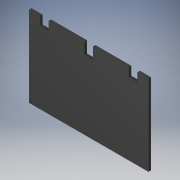
# Autodesk Inventor part: BA12
Saved by Autodesk Inventor 2017 (Build 210142000, 142)
## iProperties
Created: 2018-10-18
Part Number: BA12
Material: ABS Plastic
Document SubType Name: Modeling
Designer: Dell
Density: 1.06 g/cm^3
Appearance: Smooth - Black
Author: Dell
Autodesk Inventor part; units mm, degrees
ref_plane "YZ Plane" through (0, 0, 0) normal (1, 0, 0) x (0, 1, 0)
ref_plane "XZ Plane" through (0, 0, 0) normal (0, 1, 0) x (-1, 0, 0)
ref_plane "XY Plane" through (0, 0, 0) normal (0, 0, 1) x (1, 0, 0)
sketch "Sketch1" plane through (0, 0, 0) normal (0, 0, 1) x (1, 0, 0)
  line L0 (0, 0) -> (262.89, 0)
  line L1 (262.89, 0) -> (262.89, 355.6)
  line L2 (262.89, 355.6) -> (0, 355.6)
  line L3 (0, 355.6) -> (0, 0)
  dimension "d0" = 262.89
  dimension "d1" = 355.6
  constraints: 8 end point, 2 parallel, 1 horizontal, 1 perpendicular
  measures "d0" distance of L2.end L1.end
  measures "d1" distance of L1.end L0.end
extrude "Extrusion1" add sketch "Sketch1" along normal blind 10
sketch "Sketch3" plane through (0, 0, 10) normal (0, 0, 1) x (1, 0, 0)
  line L0 (0, 0) -> (262.89, 0) construction
  line L1 (262.89, 0) -> (262.89, 355.6) construction
  line L2 (262.89, 355.6) -> (0, 355.6) construction
  line L3 (0, 355.6) -> (0, 0) construction
  line L4 (10, 345.6) -> (252.89, 345.6) construction
  line L5 (252.89, 345.6) -> (252.89, 10) construction
  line L6 (252.89, 10) -> (10, 10) construction
  line L7 (10, 10) -> (10, 345.6) construction
  circle A0 centre (10, 345.6) radius 2.5
  circle A1 centre (10, 10) radius 2.5
  circle A2 centre (252.89, 10) radius 2.5
  circle A3 centre (252.89, 345.6) radius 2.5
  dimension "d4" = 10
  dimension "d5" = 5
  dimension "d6" = 5
  dimension "d7" = 5
  dimension "d8" = 5
  constraints: 8 end point, 4 centre point, 4 coincident, 3 other
  measures "d4" distance between parallel lines of L2 L4
  measures "d5" diameter of A0
  measures "d6" diameter of A1
  measures "d7" diameter of A2
  measures "d8" diameter of A3
extrude "Extrusion2" cut sketch "Sketch3" against normal through all
sketch "Sketch4" plane through (0, 0, 10) normal (0, 0, 1) x (1, 0, 0)
  line L0 (262.89, 355.6) -> (0, 355.6) projected
  line L1 (48.1, 355.6) -> (86.2, 355.6)
  line L2 (86.2, 355.6) -> (86.2, 317.5)
  line L3 (86.2, 317.5) -> (48.1, 317.5)
  line L4 (48.1, 317.5) -> (48.1, 355.6)
  line L5 (281.94, 355.6) -> (243.84, 355.6)
  line L6 (243.84, 355.6) -> (243.84, 304.8)
  line L7 (243.84, 304.8) -> (281.94, 304.8)
  line L8 (281.94, 304.8) -> (281.94, 355.6)
  line L9 (0, 355.6) -> (0, 0) projected
  dimension "d11" = 48.1
  dimension "d12" = 38.1
  dimension "d13" = 38.1
  dimension "d14" = 38.1
  dimension "d17" = 50.8
  constraints: 16 end point, 4 parallel, 2 horizontal, 2 perpendicular, 2 point on line, 1 midpoint
  measures "d11" distance between parallel lines of L9 L4
  measures "d12" distance between parallel lines of L8 L6
  measures "d13" distance of L3.end L1.start
  measures "d14" distance between parallel lines of L2 L4
  measures "d17" distance of L7.end L5.start
extrude "Extrusion3" cut sketch "Sketch4" against normal through all
mirror "Mirror1" about plane through (262.89, 0, 0) normal (1, 0, 0) of "Extrusion3", "Extrusion1", "Extrusion2"
body "Solid1"
